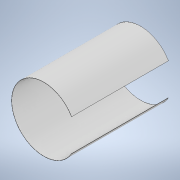
# Autodesk Inventor part: tambor
Saved by Autodesk Inventor 2021 (Build 250183000, 183)
## iProperties
Created: 2021-11-08
Part Number: tambor
Material: Genérico
Document SubType Name: Chapa
Designer: arthu
Density: 1 g/cm^3
Sheet Metal Rule: Por defecto
Appearance: Valor por defecto
Author: arthu
Autodesk Inventor part; units mm, degrees
ref_plane "YZ Plane" through (0, 0, 0) normal (1, 0, 0) x (0, 1, 0)
ref_plane "XZ Plane" through (0, 0, 0) normal (0, 1, 0) x (-1, 0, 0)
ref_plane "XY Plane" through (0, 0, 0) normal (0, 0, 1) x (1, 0, 0)
sketch "Boceto1" plane through (0, 0, 0) normal (0, 0, 1) x (1, 0, 0)
  circle A0 centre (0, 0) radius 185
  circle A1 centre (0, 0) radius 186.2
  dimension "d0" = 370
  dimension "d1" = 372.4
  constraints: 2 centre point, 2 coincident
  measures "d0" diameter of A0
  measures "d1" diameter of A1
extrude "Extrusión1" add sketch "Boceto1" along normal blind 560
sketch "Boceto3" plane through (0, 0, 560) normal (0, 0, 1) x (1, 0, 0)
  line L0 (0, 0) -> (161.2539, 93.1)
  line L1 (0, 0) -> (193.6535, 0) construction
  line L2 (0, 0) -> (161.2539, -93.1)
  line L3 (0, 0) -> (273.8674, 0) construction
  circle A0 centre (0, 0) radius 186.2 projected
  circle A1 centre (0, 0) radius 185 projected
  point P0 (160.2147, -92.5)
  point P1 (160.2147, 92.5)
  dimension "d5" = 30
  dimension "d6" = 30
  constraints: 8 end point, 2 horizontal, 2 point on circle
  measures "d5" angle of L1 L0
  measures "d6" angle of L2 L3
extrude "Extrusión2" cut sketch "Boceto3" against normal blind 1000 contours L0 A0 L2 A1 picked at (185.3292, -10.7841)
equation "\"Radio_pliegue\" = Grosor"
equation "\"Anchura_desahogo_plegado\" = Grosor"
equation "\"Profundidad_desahogo_plegado\" = 0.5 * Grosor"
equation "\"Tamaño_destalonado\" = 4 * Grosor"
equation "\"Remanente_mínimo\" = 2 * Grosor"
equation "\"Radiodetransición\" = Radio_pliegue"
equation "\"Tamaño_de_radio_de_Jacobi\" = Grosor"
equation "\"TamañoSeparación\" = Grosor"
equation "\"Grosor\" = 0.5"
